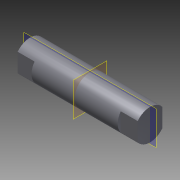
# Autodesk Inventor part: D-035
Saved by Autodesk Inventor 2015 (Build 190159000, 159)
## iProperties
Company: MARCHA TECHNOLOGY
Created: 2013-10-24
Part Number: D-035
Document SubType Name: Modeling
Designer: O.Martin
Density: 7.85 g/cm^3
Project: WITBOXprinter_K01
Material: Steel
Description: EJE CORREA X
Stock Number: 28655
Mass: 2.65111 g
Surface Area: 3.22013 cm^2
Volume: 0.337721 cm^3
Appearance: Steel
Author: O.Martin
Autodesk Inventor part; units mm, degrees
ref_plane "XY Plane" through (0, 0, 0) normal (0, 0, 1) x (1, 0, 0)
sketch "Boceto1" plane through (0, 0, 0) normal (0, 0, 1) x (1, 0, 0)
  line L0 (-9.75, 2.5) -> (9.75, 2.5)
  line L1 (9.75, 2.5) -> (9.75, 0)
  line L2 (9.75, 0) -> (-9.75, 0)
  line L3 (-9.75, 0) -> (-9.75, 2.5)
  line L4 (-9.75, 2.5) -> (-7, 2.5)
  line L5 (-7, 2.5) -> (-7, 2)
  line L6 (-7, 2) -> (-9.75, 2)
  line L7 (-9.75, 2) -> (-9.75, 2.5)
  line L8 (9.75, 2.5) -> (7, 2.5)
  line L9 (7, 2.5) -> (7, 2)
  line L10 (7, 2) -> (9.75, 2)
  line L11 (9.75, 2) -> (9.75, 2.5)
  point P0 (0, 0)
  point P1 (0, 0)
  dimension "d0" = 5
  dimension "d22" = 19.5
  dimension "d23" = 14
  dimension "d24" = 4
  constraints: 24 end point, 6 parallel, 3 horizontal, 3 perpendicular, 2 equal length, 1 coincident, 1 midpoint
  measures "d0" diameter of L0 L2
  measures "d22" distance of L1.end L2.end
  measures "d23" distance between parallel lines of L9 L5
  measures "d24" diameter of L6 L2
revolve "Revolución1" add sketch "Boceto1" angle 360 about axis through (9.75, 0, 0) along (-1, 0, 0)
sketch "Boceto3" plane through (-9.75, 0, 0) normal (-1, 0, 0) x (0, 0, 1)
  circle A0 centre (0, 0) radius 2.5 projected
  line L0 (-1.5, 2) -> (1.5, 2)
  line L1 (-1.5, -2) -> (1.5, -2)
  dimension "d27" = 4
  constraints: 4 end point, 4 point on circle, 2 parallel, 1 horizontal
  measures "d27" distance between parallel lines of L0 L1
extrude "Extrusión3" cut sketch "Boceto3" against normal blind 2.75 contours L0 A0 | A0 L1
mirror "Simetría2" about plane through (0, 0, 0) normal (1, 0, 0) of "Extrusión3"
body "Solid1"
